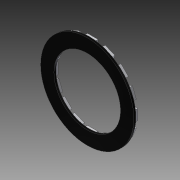
# Autodesk Inventor part: AdafruitNeoPixelRing16x
Saved by Autodesk Inventor 2014 (Build 180170000, 170)
## iProperties
Created: 2013-11-03
Part Number: AdafruitNeoPixelRing16x
Material: Generic
Document SubType Name: Modeling
Designer: blacki
Density: 1 g/cm^3
Appearance: Default
Author: blacki
Autodesk Inventor part; units mm, degrees
ref_plane "YZ Plane" through (0, 0, 0) normal (1, 0, 0) x (0, 1, 0)
ref_plane "XZ Plane" through (0, 0, 0) normal (0, 1, 0) x (-1, 0, 0)
ref_plane "XY Plane" through (0, 0, 0) normal (0, 0, 1) x (1, 0, 0)
sketch "Sketch1" plane through (0, 0, 0) normal (0, 1, 0) x (-1, 0, 0)
  circle A0 centre (0, 0) radius 22.25
  circle A1 centre (0, 0) radius 15.875
  dimension "d0" = 44.5
  dimension "d1" = 31.75
  constraints: 2 centre point, 2 coincident
  measures "d0" diameter of A0
  measures "d1" diameter of A1
extrude "Extrusion1" add sketch "Sketch1" along normal blind 1
sketch "Sketch2" plane through (0, 1, 0) normal (0, 1, 0) x (1, 0, 0)
  circle A0 centre (0, 0) radius 15.875 projected
  circle A1 centre (0, 0) radius 22.25 projected
  line L0 (-2.5, 21.5) -> (2.5, 21.5)
  line L1 (2.5, 21.5) -> (2.5, 16.5)
  line L2 (2.5, 16.5) -> (-2.5, 16.5)
  line L3 (-2.5, 16.5) -> (-2.5, 21.5)
  line L4 (0, 22.25) -> (0, 0) construction
  point P0 (0, 21.5)
  dimension "d4" = 5
  dimension "d5" = 5
  dimension "d6" = 16.5
  constraints: 10 end point, 3 parallel, 1 horizontal, 1 midpoint, 1 perpendicular, 1 point on line, 1 vertical alignment, 1 other
  measures "d4" distance of L1.end L2.end
  measures "d5" distance of L0.end L1.end
  measures "d6" distance from line of A0.centre L2
extrude "Extrusion2" add sketch "Sketch2" along normal blind 1.65 contours L0 L1 L2 L3
sketch "Sketch3" plane through (0, 2.65, 0) normal (0, 1, 0) x (1, 0, 0)
  line L0 (2.5, 21.5) -> (-2.5, 21.5) projected
  line L1 (-2.5, 16.5) -> (2.5, 16.5) projected
  circle A0 centre (0, 19) radius 1.9
  line L2 (0, 21.5) -> (0, 16.5) construction
  point P0 (0, 0)
  point P1 (0, 19)
  dimension "d9" = 3.8
  constraints: 3 midpoint, 2 end point, 1 centre point, 1 coincident
  measures "d9" diameter of A0
extrude "Extrusion3" cut sketch "Sketch3" against normal blind 0.65
chamfer "Chamfer1" distance 0.65 angle 45 1 edges at (-1.9, 2, -19)
pattern_circular "Circular Pattern1" count 16 over 360 about axis through (0, -10, 0) along (0, 1, 0) of "Extrusion3", "Extrusion2", "Chamfer1"
body "Solid1"
